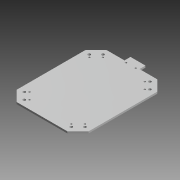
# Autodesk Inventor part: Bottom_Flame
Saved by Autodesk Inventor 2013 (Build 170138000, 138)
## iProperties
Created: 2014-02-12
Material: アルミニウム 6061
Document SubType Name: Modeling
Designer: andou
Density: 2.71 g/cm^3
Mass: 165.497 g
Surface Area: 432.933 cm^2
Volume: 61.0692 cm^3
Author: andou
Title: Bottom_Flame
Autodesk Inventor part; units mm, degrees
ref_plane "YZ Plane" through (0, 0, 0) normal (1, 0, 0) x (0, 1, 0)
ref_plane "XZ Plane" through (0, 0, 0) normal (0, 1, 0) x (-1, 0, 0)
ref_plane "XY Plane" through (0, 0, 0) normal (0, 0, 1) x (1, 0, 0)
sketch "スケッチ1" plane through (0, 0, 0) normal (0, 0, 1) x (1, 0, 0)
  line L0 (-60, 75) -> (60, 75)
  line L1 (60, 75) -> (60, -75)
  line L2 (60, -75) -> (-60, -75)
  line L3 (-60, -75) -> (-60, 75)
  line L4 (60, 92.6777) -> (77.6777, 75)
  line L5 (77.6777, 75) -> (60, 57.3223)
  line L6 (60, 57.3223) -> (42.3223, 75)
  line L7 (42.3223, 75) -> (60, 92.6777)
  line L8 (60, -57.3223) -> (77.6777, -75)
  line L9 (77.6777, -75) -> (60, -92.6777)
  line L10 (60, -92.6777) -> (42.3223, -75)
  line L11 (42.3223, -75) -> (60, -57.3223)
  line L12 (-60, -57.3223) -> (-42.3223, -75)
  line L13 (-42.3223, -75) -> (-60, -92.6777)
  line L14 (-60, -92.6777) -> (-77.6777, -75)
  line L15 (-77.6777, -75) -> (-60, -57.3223)
  line L16 (-60, 92.6777) -> (-42.3223, 75)
  line L17 (-42.3223, 75) -> (-60, 57.3223)
  line L18 (-60, 57.3223) -> (-77.6777, 75)
  line L19 (-77.6777, 75) -> (-60, 92.6777)
  point P0 (0, 0)
  dimension "d0" = 150
  dimension "d1" = 75
  dimension "d2" = 120
  dimension "d3" = 60
  dimension "d4" = 12.5
  dimension "d5" = 12.5
  dimension "d6" = 12.5
  dimension "d7" = 12.5
  constraints: 40 end point, 4 coincident, 4 point on line, 2 parallel, 1 horizontal, 1 perpendicular, 36 other
  measures "d0" distance of L2.end L0.start
  measures "d1" distance from line of point (0, 0) L2
  measures "d2" distance of L0.start L0.end
  measures "d3" distance from line of L3 point (0, 0)
  measures "d4" distance from line of L19 point (-60, 75)
  measures "d5" distance from line of L4 L0.end
  measures "d6" distance from line of L14 L2.end
  measures "d7" distance from line of L1.end L9
extrude "押し出し1" add sketch "スケッチ1" along normal blind 3
sketch "スケッチ2" plane through (0, 0, 3) normal (0, 0, 1) x (1, 0, 0)
  line L0 (77.6777, 75) -> (60, 57.3223) projected
  line L1 (60, 92.6777) -> (77.6777, 75) projected
  line L2 (42.3223, 75) -> (60, 92.6777) projected
  line L3 (-60, 92.6777) -> (-42.3223, 75) projected
  line L4 (-77.6777, 75) -> (-60, 92.6777) projected
  line L5 (-60, 57.3223) -> (-77.6777, 75) projected
  line L6 (-77.6777, -75) -> (-60, -57.3223) projected
  line L7 (-60, -92.6777) -> (-77.6777, -75) projected
  line L8 (-42.3223, -75) -> (-60, -92.6777) projected
  line L9 (60, -92.6777) -> (42.3223, -75) projected
  line L10 (77.6777, -75) -> (60, -92.6777) projected
  line L11 (60, -57.3223) -> (77.6777, -75) projected
  circle A0 centre (-46.2114, -49.8977) radius 1.5
  circle A1 centre (-34.8977, -61.2114) radius 1.5
  circle A2 centre (34.8977, -61.2114) radius 1.5
  circle A3 centre (46.2114, -49.8977) radius 1.5
  circle A4 centre (46.2114, 49.8977) radius 1.5
  circle A5 centre (34.8977, 61.2114) radius 1.5
  circle A6 centre (-34.8977, 61.2114) radius 1.5
  circle A7 centre (-46.2114, 49.8977) radius 1.5
  point P0 (0, 0)
  dimension "d10" = 3
  dimension "d12" = 40
  dimension "d13" = 40
  dimension "d14" = 4.5
  dimension "d15" = 4.5
  dimension "d16" = 40
  dimension "d17" = 40
  dimension "d18" = 40
  dimension "d19" = 40
  dimension "d20" = 40
  dimension "d21" = 40
  dimension "d22" = 4.5
  dimension "d23" = 4.5
  dimension "d24" = 4.5
  dimension "d25" = 4.5
  dimension "d26" = 4.5
  dimension "d27" = 4.5
  constraints: 8 centre point, 7 equal radius
  measures "d10" diameter of A0
  measures "d12" distance from line of A0.centre L7
  measures "d13" distance from line of L7 A1.centre
  measures "d14" distance from line of L6 A0.centre
  measures "d15" distance from line of A1.centre L8
  measures "d16" distance from line of A2.centre L10
  measures "d17" distance from line of A3.centre L10
  measures "d18" distance from line of L1 A4.centre
  measures "d19" distance from line of L1 A5.centre
  measures "d20" distance from line of L4 A7.centre
  measures "d21" distance from line of L4 A6.centre
  measures "d22" distance from line of L5 A7.centre
  measures "d23" distance from line of L3 A6.centre
  measures "d24" distance from line of L2 A5.centre
  measures "d25" distance from line of A4.centre L0
  measures "d26" distance from line of L9 A2.centre
  measures "d27" distance from line of L11 A3.centre
hole "穴1" at (34.8977, -61.2114, 3) at (46.2114, -49.8977, 3) at (-34.8977, -61.2114, 3) at (-46.2114, -49.8977, 3) at (34.8977, 61.2114, 3) at (46.2114, 49.8977, 3) at (-46.2114, 49.8977, 3) at (-34.8977, 61.2114, 3) direction (0, 0, -1) diameter 3 end through all
sketch "スケッチ3" plane through (0, 0, 3) normal (0, 0, 1) x (1, 0, 0)
  line L0 (77.6777, 75) -> (60, 57.3223) projected
  line L1 (60, 92.6777) -> (77.6777, 75) projected
  line L2 (42.3223, 75) -> (60, 92.6777) projected
  line L3 (-60, 92.6777) -> (-42.3223, 75) projected
  line L4 (-77.6777, 75) -> (-60, 92.6777) projected
  line L5 (-60, 57.3223) -> (-77.6777, 75) projected
  line L6 (-77.6777, -75) -> (-60, -57.3223) projected
  line L7 (-60, -92.6777) -> (-77.6777, -75) projected
  line L8 (-42.3223, -75) -> (-60, -92.6777) projected
  line L9 (60, -92.6777) -> (42.3223, -75) projected
  line L10 (77.6777, -75) -> (60, -92.6777) projected
  line L11 (60, -57.3223) -> (77.6777, -75) projected
  circle A0 centre (-39.1403, 65.4541) radius 2.25
  circle A1 centre (-50.4541, 54.1403) radius 2.25
  circle A2 centre (-50.4541, -54.1403) radius 2.25
  circle A3 centre (-39.1403, -65.4541) radius 2.25
  circle A4 centre (39.1403, -65.4541) radius 2.25
  circle A5 centre (50.4541, -54.1403) radius 2.25
  circle A6 centre (50.4541, 54.1403) radius 2.25
  circle A7 centre (39.1403, 65.4541) radius 2.25
  point P0 (0, 0)
  dimension "d35" = 4.5
  dimension "d37" = 4.5
  dimension "d38" = 4.5
  dimension "d39" = 34
  dimension "d40" = 34
  dimension "d41" = 4.5
  dimension "d42" = 4.5
  dimension "d43" = 34
  dimension "d44" = 34
  dimension "d45" = 34
  dimension "d46" = 4.5
  dimension "d47" = 4.5
  dimension "d48" = 34
  dimension "d49" = 34
  dimension "d50" = 34
  dimension "d51" = 4.5
  dimension "d52" = 4.5
  constraints: 8 centre point, 7 equal radius
  measures "d35" diameter of A0
  measures "d37" distance from line of L3 A0.centre
  measures "d38" distance from line of L5 A1.centre
  measures "d39" distance from line of L4 A1.centre
  measures "d40" distance from line of L4 A0.centre
  measures "d41" distance from line of L2 A7.centre
  measures "d42" distance from line of L0 A6.centre
  measures "d43" distance from line of L1 A6.centre
  measures "d44" distance from line of L1 A7.centre
  measures "d45" distance from line of L10 A5.centre
  measures "d46" distance from line of L11 A5.centre
  measures "d47" distance from line of L9 A4.centre
  measures "d48" distance from line of L10 A4.centre
  measures "d49" distance from line of L7 A3.centre
  measures "d50" distance from line of L7 A2.centre
  measures "d51" distance from line of L6 A2.centre
  measures "d52" distance from line of L8 A3.centre
hole "穴2" at (-50.4541, -54.1403, 3) at (-39.1403, -65.4541, 3) at (39.1403, 65.4541, 3) at (50.4541, 54.1403, 3) at (-50.4541, 54.1403, 3) at (-39.1403, 65.4541, 3) at (39.1403, -65.4541, 3) at (50.4541, -54.1403, 3) direction (0, 0, -1) diameter 4.5 end through all
sketch "スケッチ4" plane through (0, 0, 3) normal (0, 0, 1) x (1, 0, 0)
  line L0 (77.6777, 75) -> (60, 57.3223) projected
  line L1 (60, 92.6777) -> (77.6777, 75) projected
  line L2 (42.3223, 75) -> (60, 92.6777) projected
  line L3 (-60, 92.6777) -> (-42.3223, 75) projected
  line L4 (-77.6777, 75) -> (-60, 92.6777) projected
  line L5 (-60, 57.3223) -> (-77.6777, 75) projected
  line L6 (-77.6777, -75) -> (-60, -57.3223) projected
  line L7 (-60, -92.6777) -> (-77.6777, -75) projected
  line L8 (-42.3223, -75) -> (-60, -92.6777) projected
  line L9 (60, -92.6777) -> (42.3223, -75) projected
  line L10 (77.6777, -75) -> (60, -92.6777) projected
  line L11 (60, -57.3223) -> (77.6777, -75) projected
  line L12 (-60, -57.3223) -> (-42.3223, -75)
  line L13 (42.3223, -75) -> (60, -57.3223)
  line L14 (42.3223, 75) -> (60, 57.3223)
  line L15 (-60, 57.3223) -> (-42.3223, 75)
  point P0 (0, 0)
  dimension "d60" = 25
  dimension "d61" = 25
  dimension "d62" = 25
  dimension "d63" = 25
  constraints: 8 end point, 8 point on line, 4 perpendicular
  measures "d60" distance between parallel lines of L4 L15
  measures "d61" distance between parallel lines of L12 L7
  measures "d62" distance between parallel lines of L13 L10
  measures "d63" distance between parallel lines of L1 L14
extrude "押し出し2" cut sketch "スケッチ4" against normal blind 3
sketch "スケッチ6" plane through (-42.3223, 75, 0) normal (0, 1, 0) x (1, 0, 0)
  line L0 (84.6447, 0) -> (0, 0) projected
  line L1 (0, -3) -> (84.6447, -3) projected
  line L2 (29.8223, 0) -> (54.8223, 0)
  line L3 (54.8223, 0) -> (54.8223, -3)
  line L4 (54.8223, -3) -> (29.8223, -3)
  line L5 (29.8223, -3) -> (29.8223, 0)
  point P0 (42.3223, 0)
  dimension "d66" = 25
  dimension "d68" = 12.5
  constraints: 8 end point, 2 parallel, 2 point on line, 1 horizontal, 1 perpendicular
  measures "d66" distance of L3.end L4.end
  measures "d68" distance from line of L3 point (42.322, 0)
extrude "押し出し3" add sketch "スケッチ6" along normal blind 10
sketch "スケッチ7" plane through (0, 0, 3) normal (0, 0, 1) x (1, 0, 0)
  line L0 (-12.5, 85) -> (12.5, 85) projected
  line L1 (-12.5, 75) -> (-12.5, 85) projected
  circle A0 centre (-8, 73) radius 1.5
  circle A1 centre (8, 73) radius 1.5
  point P0 (0, 0)
  dimension "d71" = 16
  dimension "d72" = 12
  dimension "d73" = 12
  dimension "d74" = 3
  dimension "d75" = 4.5
  constraints: 2 centre point, 1 equal radius
  measures "d71" distance of A1.centre A0.centre
  measures "d72" distance from line of L0 A0.centre
  measures "d73" distance from line of L0 A1.centre
  measures "d74" diameter of A1
  measures "d75" distance from line of L1 A0.centre
hole "穴3" at (-8, 73, 3) at (8, 73, 3) direction (0, 0, -1) diameter 3 end through all
equation "\"d33\" = d26"
equation "\"d58\" = d46"
